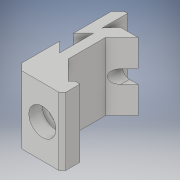
# Autodesk Inventor part: bolt_part
Saved by Autodesk Inventor 2019 (Build 230136000, 136)
## iProperties
Created: 2021-10-21
Part Number: bolt_part
Material: Genérico
Document SubType Name: Modeling
Designer: Juan M. Casillas
Density: 1 g/cm^3
Appearance: Valor por defecto
Author: Juan M. Casillas
Autodesk Inventor part; units mm, degrees
ref_plane "YZ Plane" through (0, 0, 0) normal (1, 0, 0) x (0, 1, 0)
ref_plane "XZ Plane" through (0, 0, 0) normal (0, 1, 0) x (-1, 0, 0)
ref_plane "XY Plane" through (0, 0, 0) normal (0, 0, 1) x (1, 0, 0)
sketch "Sketch1" plane through (0, 0, 0) normal (0, 1, 0) x (-1, 0, 0)
  line L0 (7.031, 15.16) -> (-6.9736, 15.16)
  line L1 (6.9783, -15.1701) -> (7.031, 15.16)
  line L2 (7.031, 15.16) -> (-7.0217, -15.14) construction
  line L3 (-6.9736, 15.16) -> (6.9783, -15.1701) construction
  line L4 (-5.5, 10.15) -> (-3.5, 10.15) construction
  line L5 (6.9783, -15.1701) -> (4.0783, -15.1701)
  line L6 (4.0783, -15.1701) -> (4.0783, -7.6701)
  line L7 (-5.5, 10.15) -> (-4, 10.15) construction
  line L8 (1.5552, -10.543) -> (4.0783, -7.6701)
  line L9 (-6.9736, 15.16) -> (-6.9736, 9.96)
  line L10 (-6.9736, 9.96) -> (-5.4736, 9.96)
  line L11 (-5.4736, 9.96) -> (-4.4736, 10.96)
  line L12 (-5.4736, 9.96) -> (-4.0594, 9.96) construction
  line L13 (-4.4736, 10.96) -> (1.1832, 5.3031)
  line L14 (1.1832, 5.3031) -> (1.1832, -5.7347)
  line L15 (1.1832, -5.7347) -> (9.1832, -5.7347) construction
  line L16 (1.1832, -5.7347) -> (-3.6251, -10.543)
  line L17 (-3.6251, -10.543) -> (1.5552, -10.543)
  point P0 (0, 0)
  point P1 (-6.5, 10.15)
  dimension "d0" = 14
  dimension "d1" = 30.3
  dimension "d11" = 2.9
  dimension "d12" = 7.5
  dimension "d25" = 41.29
  dimension "d28" = 5.2
  dimension "d29" = 1.5
  dimension "d32" = 4.2
  dimension "d33" = 8
  dimension "d38" = 6.8
  dimension "d40" = 135
  dimension "d41" = 90
  dimension "d42" = 135
  constraints: 37 end point, 8 horizontal, 2 point on line, 2 vertical, 1 equal length, 1 perpendicular
  measures "d0" distance of L1.start L2.end
  measures "d1" distance of L2.end L0.end
  measures "d11" distance of L1.start L5.end
  measures "d12" distance of L6.end L5.end
  measures "d25" angle of L8 L6
  measures "d28" distance of L0.end L9.end
  measures "d29" distance of L9.end L10.end
  measures "d32" distance from line of L0 L11.end
  measures "d33" distance of L11.end L13.end
  measures "d38" distance of L14.end L16.end
  measures "d40" angle of L13 L14
  measures "d41" angle of L13 L11
  measures "d42" angle of L16 L14
extrude "Extrusion1" add sketch "Sketch1" along normal blind 20
chamfer "Chamfer1" distance 2 angle 45 2 edges at (-7.031, 10, 15.16) (-6.9783, 10, -15.1701)
chamfer "Chamfer2" distance 1 angle 45 1 edges at (6.9736, 10, 15.16)
sketch "Sketch3" plane through (3.6251, 0, -10.543) normal (0, 0, -1) x (-1, 0, 0)
  line L0 (0, 0) -> (5.1803, 0) construction
  line L1 (5.1803, 0) -> (5.1803, 20) construction
  line L2 (0, 20) -> (5.1803, 20) construction
  line L3 (0, 0) -> (0, 20) construction
  line L4 (8.6561, 20) -> (-2.3485, 20) construction
  line L5 (5.1803, 0) -> (5.1803, 20) construction
  line L6 (5.1803, 10) -> (2.5543, 10) construction
  point P0 (3.6251, 0)
  dimension "d45" = 2.626
  constraints: 2 end point, 1 coincident, 1 horizontal, 1 midpoint
  measures "d45" distance of L6.start L6.end
hole "Hole1" at (1.0708, 10, -10.543) direction (0, 0, 1) diameter 4 end through all
sketch "Sketch4" plane through (3.6251, 0, -10.543) normal (0, 0, -1) x (-1, 0, 0)
  circle A0 centre (2.5543, 10) radius 2 construction
  line L0 (2.5543, 8) -> (2.5543, 12)
  circle A1 centre (2.5543, 10) radius 2 construction
  line L1 (2.5543, 8) -> (0, 8)
  line L2 (0, 0) -> (0, 20) projected
  line L3 (0, 8) -> (0, 12)
  line L4 (0, 12) -> (2.5543, 12)
  point P0 (3.6251, 0)
  constraints: 8 end point, 2 perpendicular, 1 horizontal, 1 point on circle, 1 point on line, 1 vertical, 1 vertical alignment, 1 other
extrude "Extrusion2" cut sketch "Sketch4" against normal blind 5
sketch "Sketch5" plane through (-5.031, 0, 15.16) normal (0, 0, 1) x (1, 0, 0)
  circle A0 centre (6.1018, 10) radius 2 projected
  point P0 (5.031, 0)
  constraints: 1 coincident
hole "Hole2" at (1.0708, 10, 15.16) direction (0, 0, -1) diameter 8 depth 4
sketch "Sketch6" plane through (0, 20, 0) normal (0, 1, 0) x (1, 0, 0)
  line L0 (6.9736, -14.16) -> (5.9736, -15.16) construction
  line L1 (6.9736, -14.16) -> (6.9736, -9.96) construction
  line L2 (6.9736, -9.96) -> (5.4736, -9.96) construction
  line L3 (5.4736, -9.96) -> (4.4736, -10.96) construction
  line L4 (4.4736, -10.96) -> (-1.1832, -5.3031) construction
  line L5 (-1.1832, -5.3031) -> (-1.1832, 5.7347) construction
  line L6 (-1.1832, 5.7347) -> (3.6251, 10.543) construction
  line L7 (3.6251, 10.543) -> (-1.5552, 10.543) construction
  line L8 (-1.5552, 10.543) -> (-4.0783, 7.6701) construction
  line L9 (-4.0783, 7.6701) -> (-4.0783, 15.1701) construction
  line L10 (-4.0783, 15.1701) -> (-4.9783, 15.1701) construction
  line L11 (-6.9817, 13.1701) -> (-4.9783, 15.1701) construction
  line L12 (-6.9817, 13.1701) -> (-7.0275, -13.16) construction
  line L13 (-5.031, -15.16) -> (-7.0275, -13.16) construction
  line L14 (-5.031, -15.16) -> (5.9736, -15.16) construction
  line L15 (-6.9817, 13.1701) -> (-7.0275, -13.16) construction
  line L16 (-7.0275, -13.16) -> (-7.0046, 0.005) construction
  line L17 (-7.0046, 0.005) -> (-4.0046, -0.0002) construction
  line L18 (-4.0046, -0.0002) -> (-4.0046, 4.9998)
  line L19 (-4.0046, -0.0002) -> (0.9954, -0.0002) construction
  line L20 (-4.0046, -0.0002) -> (-4.0046, -5.0002)
  line L21 (-4.0046, -5.0002) -> (-7.0081, -1.9967)
  line L22 (-4.0046, 4.9998) -> (-7.0011, 2.0033)
  line L23 (-7.0081, -1.9967) -> (-7.0011, 2.0033)
  point P0 (0, 0)
  dimension "d63" = 13.165
  dimension "d64" = 3
  dimension "d65" = 5
  dimension "d66" = 90
  dimension "d67" = 5
  dimension "d68" = 45
  dimension "d69" = 45
  constraints: 16 end point, 3 point on line, 2 perpendicular, 2 vertical, 1 horizontal
  measures "d63" distance of L12.end L16.end
  measures "d64" distance of L16.end L17.end
  measures "d65" distance of L17.end L18.end
  measures "d66" angle of L19 L18
  measures "d67" distance of L17.end L20.end
  measures "d68" angle of L20 L21
  measures "d69" angle of L18 L22
extrude "Extrusion3" cut sketch "Sketch6" against normal through all
equation "\"d42\" = d40"
equation "\"d69\" = d68"
body "Solid1"
